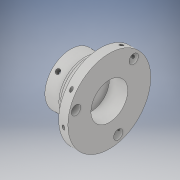
# Autodesk Inventor part: Pen Interface V2
Saved by Autodesk Inventor 2019 (Build 230136000, 136)
## iProperties
Created: 2019-06-10
Part Number: Pen Interface V2
Material: Generic
Document SubType Name: Modeling
Designer: Matthew XPS
Density: 1 g/cm^3
Appearance: Default
Author: Matthew XPS
Autodesk Inventor part; units mm, degrees
ref_plane "YZ Plane" through (0, 0, 0) normal (1, 0, 0) x (0, 1, 0)
ref_plane "XZ Plane" through (0, 0, 0) normal (0, 1, 0) x (-1, 0, 0)
ref_plane "XY Plane" through (0, 0, 0) normal (0, 0, 1) x (1, 0, 0)
sketch "Sketch2" plane through (0, 0, 0) normal (1, 0, 0) x (0, 1, 0)
  circle A0 centre (0, 0) radius 10
  circle A1 centre (0, 0) radius 22
  line L0 (0, 0) -> (7.0711, -7.0711)
  line L1 (0, 0) -> (10, 0) construction
  circle A2 centre (7.0711, -7.0711) radius 1.5
  line L2 (0, 0) -> (10.8294, 10.8294)
  line L3 (0, 0) -> (15.315, 0) construction
  circle A3 centre (-7.0711, 7.0711) radius 1.5
  dimension "d3" = 20
  dimension "d4" = 44
  dimension "d16" = 10
  dimension "d17" = 45
  dimension "d18" = 3
  dimension "d19" = 45
  constraints: 8 end point, 4 centre point, 3 coincident, 2 equal length, 2 horizontal, 1 symmetric about line, 1 other
  measures "d3" diameter of A0
  measures "d4" diameter of A1
  measures "d16" distance of L0.start L0.end
  measures "d17" angle of L0 L1
  measures "d18" diameter of A2
  measures "d19" angle of L3 L2
extrude "Extrusion1" add sketch "Sketch2" along normal blind 12 contours A2 A0 | A0 L0 A2 | A3 A0 | A0 A3 | A0 A2 L0 | A1
sketch "Sketch4" plane through (0, 0, 0) normal (1, 0, 0) x (0, 0, -1)
  circle A0 centre (0, 0) radius 15.75
  circle A1 centre (15.75, 0) radius 2.55
  dimension "d9" = 31.5
  dimension "d10" = 5.1
  constraints: 1 centre point, 1 coincident, 1 horizontal alignment, 2 other
  measures "d10" diameter of A1
extrude "Extrusion3" cut sketch "Sketch4" along normal blind 30 contours A0 A1 | A0 A1 picked at (14.9184, -0.4924) picked at (16.4994, -0.6699)
sketch "Sketch5" plane through (12, 0, 0) normal (1, 0, 0) x (0, 0, -1)
  circle A0 centre (15.75, 0) radius 2.55 projected
  circle A1 centre (15.75, 0) radius 4.5
  point P0 (0, 0)
  dimension "d20" = 9
  constraints: 1 centre point, 1 coincident
  measures "d20" diameter of A1
extrude "Extrusion4" cut sketch "Sketch5" against normal blind 6
pattern_circular "Circular Pattern1" count 4 over 360 about axis through (-10, 0, 0) along (1, 0, 0) of "Extrusion3", "Extrusion4"
sketch "Sketch6" plane through (12, 0, 0) normal (1, 0, 0) x (0, 0, -1)
  line L0 (0, 0) -> (15.5563, 15.5563)
  line L1 (0, 0) -> (22, 0) construction
  dimension "d23" = 22
  dimension "d24" = 45
  constraints: 4 end point, 1 equal length, 1 horizontal
  measures "d23" distance of L0.start L0.end
  measures "d24" angle of L1 L0
ref_plane "Work Plane1" through (12, 15.5563, -15.5563) normal (0, 0.7071068, -0.7071068) x (-1, 0, 0)
sketch "Sketch7" plane through (12, 15.5563, -15.5563) normal (0, 0.7071068, -0.7071068) x (-1, 0, 0)
  line L0 (0, 22) -> (0, -22) projected
  line L1 (0, 0) -> (12, 0)
  circle A0 centre (6, 0) radius 2.6
  dimension "d25" = 5.2
  constraints: 2 end point, 2 midpoint, 1 centre point, 1 horizontal
  measures "d25" diameter of A0
extrude "Extrusion5" cut sketch "Sketch7" against normal blind 10
ref_plane "Work Plane2" through (12, 0, 0) normal (0, 0.7071068, -0.7071068) x (-1, 0, 0)
mirror "Mirror1" about plane through (12, 0, 0) normal (0, 0.7071068, -0.7071068) of "Extrusion5"
sketch "Sketch8" plane through (0, 0, 0) normal (1, 0, 0) x (0, 1, 0)
  circle A0 centre (-15.75, 0) radius 4.5 projected
  circle A1 centre (0, 15.75) radius 4.5 projected
  circle A2 centre (15.75, 0) radius 4.5 projected
  circle A3 centre (0, -15.75) radius 4.5 projected
  circle A4 centre (0, 0) radius 22 projected
  arc A5 (8.0492, -5.9338) -> (5.9338, -8.0492) centre (7.0711, -7.0711) ccw projected
  arc A6 (-8.0492, 5.9338) -> (5.9338, -8.0492) centre (0, 0) ccw projected
  arc A7 (-8.0492, 5.9338) -> (-5.9338, 8.0492) centre (-7.0711, 7.0711) ccw projected
  arc A8 (8.0492, -5.9338) -> (-5.9338, 8.0492) centre (0, 0) ccw projected
  arc A9 (-7.9786, 5.5166) -> (-5.5166, 7.9786) centre (-7.0711, 7.0711) ccw
  arc A10 (-7.9786, 5.5166) -> (5.5166, -7.9786) centre (0, 0) ccw
  arc A11 (7.9786, -5.5166) -> (5.5166, -7.9786) centre (7.0711, -7.0711) ccw
  arc A12 (7.9786, -5.5166) -> (-5.5166, 7.9786) centre (0, 0) ccw
  dimension "d28" = 0.3
  constraints: 8 point on circle, 4 centre point, 3 other
  measures "d28" radial gap between concentric circles of A8 A12
extrude "Extrusion6" add sketch "Sketch8" along normal blind 12 separate body contours A9 A12 A11 A10
sketch "Sketch9" plane through (0, 0, 0) normal (1, 0, 0) x (0, 1, 0)
  circle A0 centre (0, 0) radius 22 projected
  circle A1 centre (0, 0) radius 28
  circle A2 centre (0, 0) radius 22.25
  dimension "d31" = 6
  dimension "d34" = 0.25
  constraints: 2 centre point
  measures "d31" radial gap between concentric circles of A0 A1
  measures "d34" radial gap between concentric circles of A0 A2
extrude "Extrusion7" add sketch "Sketch9" along normal blind 12 contours A1 bodies 2
sketch "Sketch11" plane through (12, 0, 0) normal (1, 0, 0) x (0, 0, -1)
  line L0 (0, 0) -> (19.799, 19.799)
  circle A0 centre (0, 0) radius 28 projected
  line L1 (0, 0) -> (28, 0) construction
  dimension "d35" = 45
  constraints: 4 end point, 1 equal length, 1 horizontal, 2 other
  measures "d35" angle of L1 L0
ref_plane "Work Plane3" through (12, 19.799, -19.799) normal (0, 0.7071068, -0.7071068) x (-1, 0, 0)
sketch "Sketch12" plane through (12, 19.799, -19.799) normal (0, 0.7071068, -0.7071068) x (-1, 0, 0)
  line L0 (12, 0) -> (0, 0)
  circle A0 centre (6, 0) radius 2.5
  dimension "d36" = 12
  dimension "d37" = 5
  constraints: 2 end point, 1 centre point, 1 horizontal, 1 midpoint
  measures "d36" distance of L0.start L0.end
  measures "d37" diameter of A0
extrude "Extrusion8" cut sketch "Sketch12" against normal blind 10 bodies 2
thread "Thread1"
mirror "Mirror2" about plane through (12, 0, 0) normal (0, 0.7071068, -0.7071068) of "Extrusion8" bodies 2
sketch "Sketch13" plane through (12, 0, 0) normal (1, 0, 0) x (0, 0, -1)
  circle A0 centre (0, 0) radius 28 projected
  circle A1 centre (0, 0) radius 28 projected
extrude "Extrusion9" add sketch "Sketch13" along normal blind 5 bodies 2
sketch "Sketch14" plane through (0, 0, 0) normal (0, 1, 0) x (-1, 0, 0)
  line L0 (-17, 28) -> (-17, -28) projected
  line L1 (-17, 0) -> (-17, -28)
  line L2 (-17, 0) -> (-32, 0)
  line L3 (-17, 0) -> (-2, 0) construction
  line L4 (-32, 0) -> (-32, -45)
  line L5 (-32, 0) -> (13, 0) construction
  line L6 (-32, -45) -> (-17, -28)
  line L7 (12, 0) -> (-33.5, 0) projected
  point P0 (0, 0)
  dimension "d44" = 15
  dimension "d45" = 180
  dimension "d46" = 45
  dimension "d47" = 90
  constraints: 12 end point, 3 horizontal, 2 equal length, 2 vertical, 1 midpoint
  measures "d44" distance of L1.start L2.end
  measures "d45" angle of L2 L3
  measures "d46" distance of L2.end L4.end
  measures "d47" angle of L4 L5
revolve "Revolution1" add sketch "Sketch14" angle 360 about axis through (-10, 0, 0) along (1, 0, 0) bodies 2
mirror "Mirror3" about plane through (0, 0, 0) normal (0, 0, 1) of "Extrusion8", "Mirror2" bodies 2
fillet "Fillet1" radius 4 1 edges at (17, 0, 28)
fillet "Fillet2" radius 0.4 2 edges at (8.2998, -19.0938, 20.4799) (8.2998, 20.4799, -19.0938)
sketch "Sketch15" plane through (32, 0, 0) normal (1, 0, 0) x (0, 0, -1)
  circle A0 centre (0, 0) radius 45 projected
extrude "Extrusion10" add sketch "Sketch15" along normal blind 10 bodies 2
sketch "Sketch17" plane through (42, 0, 0) normal (1, 0, 0) x (0, 0, -1)
  line L0 (0, 0) -> (26.5165, 26.5165)
  line L1 (0, 0) -> (37.5, 0) construction
  circle A0 centre (26.5165, 26.5165) radius 5.05
  dimension "d53" = 37.5
  dimension "d54" = 45
  dimension "d55" = 10.1
  constraints: 4 end point, 1 centre point, 1 coincident, 1 equal length, 1 horizontal
  measures "d53" distance of L0.start L0.end
  measures "d54" angle of L1 L0
  measures "d55" diameter of A0
extrude "Extrusion11" cut sketch "Sketch17" against normal blind 10 bodies 2
sketch "Sketch18" plane through (42, 0, 0) normal (1, 0, 0) x (0, 0, -1)
  line L0 (8.4754, 8.8972) -> (31.6082, 32.03)
  circle A0 centre (0, 0) radius 45 projected
  line L1 (8.4754, 8.8972) -> (41.1901, 8.8972) construction
  dimension "d58" = 45
  constraints: 4 end point, 1 equal length, 1 horizontal, 2 other
  measures "d58" angle of L1 L0
ref_plane "Work Plane4" through (42, 32.03, -31.6082) normal (0, 0.711778, -0.7024045) x (-1, 0, 0)
sketch "Sketch19" plane through (42, 32.03, -31.6082) normal (0, 0.711778, -0.7024045) x (-1, 0, 0)
  line L0 (10, -5.2986) -> (10, 4.8014) projected
  line L1 (10, -2.0663) -> (5, -2.0663)
  line L2 (0, 45) -> (0, -45) projected
  line L3 (10, -2.0663) -> (15, -2.0663) construction
  point P0 (42, 0)
  dimension "d59" = 5
  dimension "d60" = 180
  constraints: 4 end point, 2 horizontal, 1 collinear, 1 point on line, 1 other
  measures "d59" distance of L1.start L1.end
  measures "d60" angle of L1 L3
ref_plane "Work Plane5" through (37, 26.5165, -26.5165) normal (1, 0, 0) x (0, 0, -1)
sketch "Sketch22" plane through (37, 26.5165, -26.5165) normal (1, 0, 0) x (0, 0, -1)
  line L0 (0, 0) -> (-20, 34.641)
  line L1 (0, 0) -> (40, 0) construction
  circle A0 centre (0, 0) radius 5.05 projected
  line L2 (0, 0) -> (34.641, -20)
  line L3 (0, 0) -> (40, 0) construction
  point P0 (-26.5165, -26.5165)
  dimension "d69" = 40
  dimension "d70" = 120
  dimension "d78" = 40
  dimension "d79" = 30
  constraints: 8 end point, 2 equal length, 2 horizontal
  measures "d69" distance of L0.start L0.end
  measures "d70" angle of L1 L0
  measures "d78" distance of L2.start L2.end
  measures "d79" angle of L2 L3
ref_plane "Work Plane6" through (37, 61.1575, -6.5165) normal (0, 0.8660254, 0.5) x (-1, 0, 0)
sketch "Sketch23" plane through (37, 61.1575, -6.5165) normal (0, 0.8660254, 0.5) x (-1, 0, 0)
  point P0 (37, 36.2222)
sketch "Sketch24" plane through (37, 61.1575, -6.5165) normal (0, 0.8660254, 0.5) x (-1, 0, 0)
  circle A0 centre (0, 0) radius 1.5
  point P0 (37, 36.2222)
  dimension "d71" = 3
  constraints: 1 centre point
  measures "d71" diameter of A0
sweep "Sweep1" cut profiles "Sketch24" path "Sketch22" bodies 2 path curves L0
ref_plane "Work Plane7" through (37, 26.5165, -26.5165) normal (0, 0.8660254, 0.5) x (-1, 0, 0)
thread "Thread3"
sketch "Sketch25" plane through (37, 26.5165, -26.5165) normal (1, 0, 0) x (0, 0, -1)
  point P0 (-26.5165, -26.5165)
sketch "Sketch26" plane through (37, 26.5165, -26.5165) normal (1, 0, 0) x (0, 0, -1)
  circle A0 centre (0, 0) radius 5.05 projected
  point P0 (-26.5165, -26.5165)
sketch "Sketch27" plane through (37, 26.5165, -26.5165) normal (1, 0, 0) x (0, 0, -1)
  line L0 (15.3855, -0.6466) -> (45.3855, -0.6466) construction
  line L1 (0, 0) -> (-17.9949, 17.9949)
  line L2 (0, 0) -> (25.4486, 0) construction
  point P0 (-26.5165, -26.5165)
  dimension "d82" = 135
  constraints: 6 end point, 2 horizontal, 1 equal length
  measures "d82" angle of L2 L1
ref_plane "Work Plane10" through (37, 26.5165, -26.5165) normal (0, 0.7071068, 0.7071068) x (-1, 0, 0)
mirror "Mirror4" about plane through (37, 26.5165, -26.5165) normal (0, 0.7071068, 0.7071068) of "Sweep1" bodies 2
pattern_circular "Circular Pattern2" count 3 over 360 about axis through (-10, 0, 0) along (1, 0, 0) of "Extrusion11", "Sweep1", "Mirror4" bodies 2
sketch "Sketch28" plane through (42, 0, 0) normal (1, 0, 0) x (0, 0, -1)
  circle A0 centre (0, 0) radius 20
  dimension "d83" = 40
  constraints: 1 centre point, 1 coincident
  measures "d83" diameter of A0
extrude "Extrusion13" cut sketch "Sketch28" against normal blind 20 bodies 2
body "Solid1"
body "Solid2"
